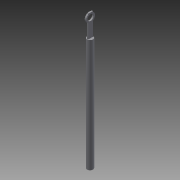
# Autodesk Inventor part: Rod
Saved by Autodesk Inventor 2015 SP1 (Build 190203100, 203)
## iProperties
Created: 2016-02-02
Part Number: Rod
Material: Generic
Document SubType Name: Modeling
Designer: tuttlem
Density: 1 g/cm^3
Appearance: Default
Author: tuttlem
Autodesk Inventor part; units mm, degrees
ref_plane "YZ Plane" through (0, 0, 0) normal (1, 0, 0) x (0, 1, 0)
ref_plane "XZ Plane" through (0, 0, 0) normal (0, 1, 0) x (-1, 0, 0)
ref_plane "XY Plane" through (0, 0, 0) normal (0, 0, 1) x (1, 0, 0)
sketch "Sketch1" plane through (0, 0, 0) normal (1, 0, 0) x (0, 1, 0)
  line L0 (-11.2229, 4.9257) -> (471.3771, 4.9257)
  line L1 (471.3771, 4.9257) -> (471.3771, -7.7743)
  line L2 (471.3771, -7.7743) -> (-11.2229, -7.7743)
  line L3 (-11.2229, -7.7743) -> (-11.2229, 4.9257)
  point P0 (0, 0)
  dimension "d0" = 482.6
  constraints: 8 end point, 2 parallel, 1 horizontal, 1 perpendicular
  measures "d0" distance of L1.end L2.end
revolve "Revolution1" add sketch "Sketch1" angle 360 about axis through (0, -11.2229, 4.9257) along (0, 1, 0)
sketch "Sketch2" plane through (0, 471.3771, 4.9257) normal (0, 1, 0) x (1, 0, 0)
  line L0 (-2.5588, -10.1161) -> (2.6183, -10.1161)
  line L1 (2.6183, -10.1161) -> (2.6183, 10.1161)
  line L2 (2.6183, 10.1161) -> (-2.5588, 10.1161)
  line L3 (-2.5588, 10.1161) -> (-2.5588, -10.1161)
  line L4 (-2.5588, 0) -> (2.6183, 0)
  point P0 (0, 4.9257)
  constraints: 10 end point, 2 midpoint, 2 parallel, 1 horizontal, 1 perpendicular
extrude "Extrusion1" add sketch "Sketch2" along normal blind 95.25
sketch "Sketch3" plane through (2.6183, 471.3771, 15.0418) normal (1, 0, 0) x (0, 0, -1)
  line L0 (20.2322, 0) -> (0, 0) projected
  line L1 (20.2322, 0) -> (20.2322, 95.25) projected
  line L2 (0, 95.25) -> (20.2322, 95.25) projected
  line L3 (0, 0) -> (0, 95.25) projected
  line L4 (-2.5839, 0) -> (22.8161, 0) projected
  line L5 (10.1161, 0) -> (10.1161, 76.2)
  circle A0 centre (10.1161, 76.2) radius 12.7
  circle A1 centre (10.1161, 76.2) radius 19.05
  point P0 (15.0418, -471.3771)
  dimension "d10" = 76.2
  dimension "d11" = 25.4
  dimension "d12" = 38.1
  constraints: 2 centre point, 2 coincident, 2 end point, 1 midpoint, 1 vertical
  measures "d10" distance of L5.start L5.end
  measures "d11" diameter of A0
  measures "d12" diameter of A1
extrude "Extrusion2" add sketch "Sketch3" against normal blind 6.35 contours A1 L5 A0 L1 | L1 A0 A1 | A1 L3 A0 L5 | A1 L3 A0 | A0 L3 A1 L1
sketch "Sketch4" plane through (2.6183, 471.3771, 15.0418) normal (1, 0, 0) x (0, 0, -1)
  line L0 (20.2322, 68.5218) -> (20.2322, 83.8782) projected
  arc A0 (20.2322, 68.5218) -> (20.2322, 83.8782) centre (10.1161, 76.2) ccw projected
  arc A1 (20.2322, 60.0579) -> (20.2322, 92.3421) centre (10.1161, 76.2) ccw projected
  line L1 (20.2322, 92.3421) -> (20.2322, 95.25) projected
  line L2 (0, 95.25) -> (20.2322, 95.25) projected
  line L3 (0, 92.3421) -> (0, 95.25) projected
  arc A2 (0, 92.3421) -> (0, 60.0579) centre (10.1161, 76.2) ccw projected
  line L4 (0, 0) -> (0, 60.0579) projected
  line L5 (20.2322, 0) -> (0, 0) projected
  line L6 (20.2322, 0) -> (20.2322, 60.0579) projected
  arc A3 (0, 83.8782) -> (0, 68.5218) centre (10.1161, 76.2) ccw projected
  line L7 (0, 68.5218) -> (0, 83.8782) projected
  arc A4 (0, 83.8782) -> (0, 68.5218) centre (10.1161, 76.2) ccw projected
  arc A5 (20.2322, 83.8782) -> (0, 83.8782) centre (10.1161, 76.2) ccw projected
  arc A6 (20.2322, 68.5218) -> (20.2322, 83.8782) centre (10.1161, 76.2) ccw projected
  arc A7 (0, 68.5218) -> (20.2322, 68.5218) centre (10.1161, 76.2) ccw projected
  circle A8 centre (10.1161, 76.2) radius 12.7
  point P0 (15.0418, -471.3771)
  constraints: 1 centre point, 1 coincident
extrude "Extrusion3" cut sketch "Sketch4" against normal blind 6.35 contours A7 L7 A5 L0 | L0 A0 | A3 L7
body "Solid1"
